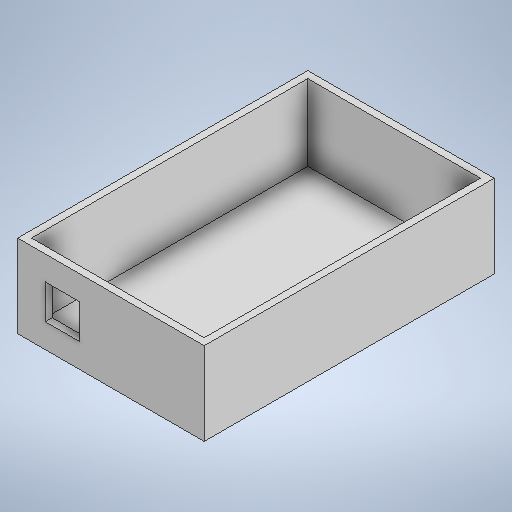
# Autodesk Inventor part: case
Saved by Autodesk Inventor 2025.1 (Build 291241000, 241)
## iProperties
Created: 2024-11-27
Part Number: case
Material: 일반
Document SubType Name: Modeling
Designer: goode
Density: 1 g/cm^3
Appearance: 기본값
Author: goode
Autodesk Inventor part; units mm, degrees
ref_plane "YZ Plane" through (0, 0, 0) normal (1, 0, 0) x (0, 1, 0)
ref_plane "XZ Plane" through (0, 0, 0) normal (0, 1, 0) x (-1, 0, 0)
ref_plane "XY Plane" through (0, 0, 0) normal (0, 0, 1) x (1, 0, 0)
sketch "스케치1" plane through (0, 0, 0) normal (0, 1, 0) x (-1, 0, 0)
  line L0 (0, 0) -> (-54, 0)
  line L1 (-54, 0) -> (-54, -84)
  line L2 (-54, -84) -> (0, -84)
  line L3 (0, -84) -> (0, 0)
  line L4 (0, 0) -> (0, -2)
  line L5 (0, -2) -> (-2, -2)
  line L6 (-54, -84) -> (-54, -82)
  line L7 (-54, -82) -> (-52, -82)
  line L8 (-2, -2) -> (-52, -2)
  line L9 (-52, -2) -> (-52, -82)
  line L10 (-52, -82) -> (-2, -82)
  line L11 (-2, -82) -> (-2, -2)
  dimension "d0" = 54
  dimension "d1" = 84
  dimension "d2" = 2
  dimension "d3" = 2
  dimension "d4" = 2
  dimension "d5" = 2
  constraints: 24 end point, 4 parallel, 4 perpendicular, 2 horizontal, 2 point on line
  measures "d0" distance of L2.end L1.end
  measures "d1" distance of L1.end L0.end
  measures "d2" distance of L0.start L4.end
  measures "d3" distance of L4.end L5.end
  measures "d4" distance of L1.end L6.end
  measures "d5" distance of L6.end L7.end
extrude "돌출1" add sketch "스케치1" along normal blind 22 contours L3 L5 L8 L9 L7 L1 L0 | L3 L2 L1 L7 L10 L11 L5
extrude "돌출2" add sketch "스케치1" against normal blind 2
sketch "스케치2" plane through (0, 22, 0) normal (0, 0, 1) x (1, 0, 0)
  line L0 (0, -22) -> (7, -22)
  line L1 (0, -22) -> (7, -22) construction
  line L2 (7, -22) -> (8, -22)
  line L3 (8, -22) -> (8, -7)
  line L4 (8, -7) -> (18, -7)
  line L5 (18, -7) -> (18, -22)
  line L6 (18, -22) -> (8, -22)
  line L7 (8, -22) -> (18, -22)
  line L8 (18, -22) -> (18, -17)
  line L9 (18, -17) -> (8, -17)
  line L10 (8, -17) -> (8, -22)
  point P0 (8, -17)
  dimension "d10" = 7
  dimension "d11" = 0
  dimension "d12" = 1
  dimension "d13" = 15
  dimension "d14" = 10
  dimension "d15" = 5
  constraints: 22 end point, 5 perpendicular, 3 horizontal, 3 point on line, 2 parallel, 1 collinear
  measures "d10" distance of L0.start L0.end
  measures "d11" distance between parallel lines of L0 L1
  measures "d12" distance of L0.end L2.end
  measures "d13" distance of L2.end L3.end
  measures "d14" distance of L3.end L4.end
  measures "d15" distance of L8.end L7.end
extrude "돌출3" cut sketch "스케치2" against normal blind 2 contours L3 L4 L5 L9
